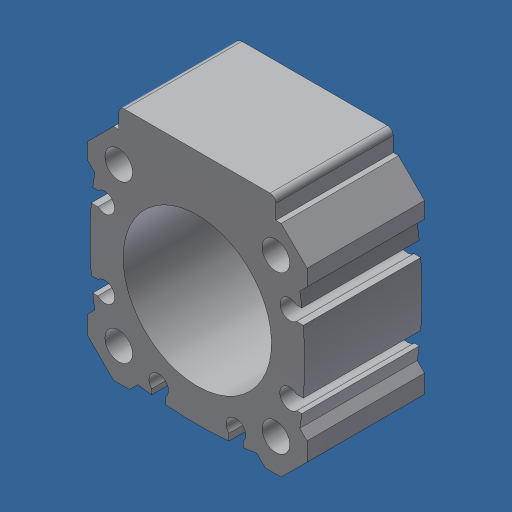
# Autodesk Inventor part: EXTRUSION, CYLINDER, ALUMINIUM, PHD, 32MM
Saved by Autodesk Inventor 2024.3 (Build 283343000, 343)
## iProperties
Manager: _
Category: _
Shininess: 64.0
Angle Display Precision: 2
Document Length Units: 11269
Document Angle Units: 11279
Document Time Units: 11290
Document Mass Units: 11286
Document Length Units Precision: 3
Document Angle Units Precision: 2
Part Number: EXTRUSION, CYLINDER, ALUMINIUM, PHD, 32MM
Material: Extrusion, Aluminum, PHD, 32MM
Document SubType Name: Modeling
Created: 2023-11-08
Designer: -
Manufacturer: Standard
Standards Organization: Custom
Checked By: 00
Engr Approved By: _
User Status: Work In Process
Description: EXTRUSION, CYLINDER, ALUMINIUM, PHD, 32MM
Density: 2.71 g/cm^3
Mass: 85.3878 g
Surface Area: 132.066 cm^2
Volume: 31.5084 cm^3
Mfg Approved By: Stephen.Oerton
Appearance: Aluminum - Flat
ILogicPurgeVersion: 2.2.20.20
OnSaveVersion: 2.2.20.20
Density: 0.0
Volumn: 0.0
Area: 0.0
PropertySet Name: Model Information
Control State: 0
Master: False
Checked Out: False
CN_MASS: 0.09
CN_SERVICEABLE: _
CL_runCount: 0
FIRST_DESCRIPTION: _
SECOND_DESCRIPTION: _
THIRD_DESCRIPTION: _
ModelCat: Uncategorized
Revision Number: A
Subject: _
Author: -
Keywords: -
Autodesk Inventor part; units mm, degrees
ref_plane "YZ Plane" through (0, 0, 0) normal (1, 0, 0) x (0, 1, 0)
ref_plane "XZ Plane" through (0, 0, 0) normal (0, 1, 0) x (-1, 0, 0)
ref_plane "XY Plane" through (0, 0, 0) normal (0, 0, 1) x (1, 0, 0)
sketch "Sketch1" plane through (0, 0, 0) normal (0, 0, 1) x (1, 0, 0)
  arc A0 (0, 16.053) -> (0, -16.053) centre (0, 0) ccw
  arc A1 (-15.7355, 27.991) -> (-17.0055, 26.721) centre (-15.7355, 26.721) ccw
  line L0 (-17.0055, 26.721) -> (-17.0055, 23.52)
  line L1 (-17.0055, 23.52) -> (-18.1469, 23.52)
  line L2 (0, 78.3044) -> (0, -31.8793) projected
  line L3 (-15.7355, 27.991) -> (0, 27.991)
  line L4 (-18.1469, 23.52) -> (-23.75, 17.9169)
  line L5 (-23.75, 17.9169) -> (-23.75, 14.428)
  line L6 (-23.75, 14.428) -> (-22.174, 12.852)
  line L7 (-22.6105, 9.8935) -> (-21.4771, 9.8935)
  arc A2 (-21.4771, 6.8205) -> (-21.4771, 9.8935) centre (-20.015, 8.357) ccw
  line L8 (-22.942, 6.8205) -> (-21.4771, 6.8205)
  arc A3 (-22.174, 12.852) -> (-22.6105, 9.8935) centre (54.6936, 0) ccw
  arc A4 (-21.544, -9.8935) -> (-21.544, -6.8205) centre (-20.015, -8.357) ccw
  line L9 (-22.942, -6.8205) -> (-21.544, -6.8205)
  line L10 (-22.6105, -9.8935) -> (-21.544, -9.8935)
  arc A5 (-22.942, 6.8205) -> (-22.942, -6.8205) centre (54.6936, 0) ccw
  arc A6 (-22.6105, -9.8935) -> (-22.174, -12.852) centre (54.6936, 0) ccw
  line L11 (-22.174, -12.852) -> (-23.75, -14.428)
  line L12 (-23.75, -14.428) -> (-23.75, -18.4059)
  line L13 (-23.75, -18.4059) -> (-18.1469, -24.009)
  line L14 (-18.1469, -24.009) -> (-14.687, -24.009)
  line L15 (-14.687, -24.009) -> (-12.852, -22.174)
  arc A7 (-6.8205, -21.4771) -> (-9.8935, -21.4771) centre (-8.357, -20.015) ccw
  line L16 (-9.8935, -21.4771) -> (-9.8935, -22.6105)
  line L17 (-6.8205, -21.4771) -> (-6.8205, -22.942)
  arc A8 (-12.852, -22.174) -> (-9.8935, -22.6105) centre (0, 54.6936) ccw
  arc A9 (-6.8205, -22.942) -> (0, -23.241) centre (0, 54.6936) ccw
  circle A10 centre (-17, -17) radius 3
  circle A11 centre (-17, 17) radius 3
  arc A12 (0, -16.053) -> (0, 16.053) centre (0, 0) ccw
  arc A13 (17.0055, 26.721) -> (15.7355, 27.991) centre (15.7355, 26.721) ccw
  line L18 (17.0055, 26.721) -> (17.0055, 23.52)
  line L19 (17.0055, 23.52) -> (18.1469, 23.52)
  line L20 (15.7355, 27.991) -> (0, 27.991)
  line L21 (18.1469, 23.52) -> (23.75, 17.9169)
  line L22 (23.75, 17.9169) -> (23.75, 14.428)
  line L23 (23.75, 14.428) -> (22.174, 12.852)
  line L24 (22.6105, 9.8935) -> (21.4771, 9.8935)
  arc A14 (21.4771, 9.8935) -> (21.4771, 6.8205) centre (20.015, 8.357) ccw
  line L25 (22.942, 6.8205) -> (21.4771, 6.8205)
  arc A15 (22.6105, 9.8935) -> (22.174, 12.852) centre (-54.6936, 0) ccw
  arc A16 (21.544, -6.8205) -> (21.544, -9.8935) centre (20.015, -8.357) ccw
  line L26 (22.942, -6.8205) -> (21.544, -6.8205)
  line L27 (22.6105, -9.8935) -> (21.544, -9.8935)
  arc A17 (22.942, -6.8205) -> (22.942, 6.8205) centre (-54.6936, 0) ccw
  arc A18 (22.174, -12.852) -> (22.6105, -9.8935) centre (-54.6936, 0) ccw
  line L28 (22.174, -12.852) -> (23.75, -14.428)
  line L29 (23.75, -14.428) -> (23.75, -18.4059)
  line L30 (23.75, -18.4059) -> (18.1469, -24.009)
  line L31 (18.1469, -24.009) -> (14.687, -24.009)
  line L32 (14.687, -24.009) -> (12.852, -22.174)
  arc A19 (9.8935, -21.4771) -> (6.8205, -21.4771) centre (8.357, -20.015) ccw
  line L33 (9.8935, -21.4771) -> (9.8935, -22.6105)
  line L34 (6.8205, -21.4771) -> (6.8205, -22.942)
  arc A20 (9.8935, -22.6105) -> (12.852, -22.174) centre (0, 54.6936) ccw
  arc A21 (0, -23.241) -> (6.8205, -22.942) centre (0, 54.6936) ccw
  circle A22 centre (17, -17) radius 3
  circle A23 centre (17, 17) radius 3
  arc A24 (22.174, -12.852) -> (22.6105, -9.8935) centre (-54.6936, 0) ccw
  arc A25 (22.942, -6.8205) -> (22.942, 6.8205) centre (-54.6936, 0) ccw
  dimension "d0" = 54.6936
  dimension "d2" = 54.6936
  dimension "d6" = 32.106
  dimension "d8" = 2.54
  dimension "d10" = 15.7355
  dimension "d11" = 26.721
  dimension "d12" = 18.1469
  dimension "d13" = 23.52
  dimension "d14" = 135
  dimension "d15" = 17.9169
  dimension "d16" = 3.4889
  dimension "d17" = 135
  dimension "d18" = 22.174
  dimension "d19" = 9.8935
  dimension "d22" = 22.6105
  dimension "d23" = 20.015
  dimension "d24" = 8.357
  dimension "d25" = 4.242
  dimension "d26" = 6.8205
  dimension "d27" = 8.357
  dimension "d28" = 4.3354
  dimension "d29" = 6.8205
  dimension "d30" = 9.8935
  dimension "d31" = 77.9346
  dimension "d32" = 22.174
  dimension "d33" = 12.852
  dimension "d34" = 45
  dimension "d35" = 14.428
  dimension "d37" = 18.4059
  dimension "d38" = 135
  dimension "d39" = 24.009
  dimension "d41" = 135
  dimension "d42" = 14.687
  dimension "d43" = 20.015
  dimension "d44" = 8.357
  dimension "d45" = 4.242
  dimension "d46" = 9.8935
  dimension "d47" = 6.8205
  dimension "d48" = 77.9346
  dimension "d49" = 77.9346
  dimension "d50" = 17
  dimension "d51" = 17
  dimension "d52" = 6
  dimension "d53" = 17
  dimension "d54" = 6
  constraints: 68 end point, 42 point on circle, 33 symmetric about line, 26 centre point, 6 perpendicular, 5 parallel, 4 point on line, 3 vertical alignment, 2 horizontal alignment, 2 tangent, 1 coincident, 1 horizontal, 29 other
  measures "d0" distance of A3.centre point (0, 0)
  measures "d2" distance of A8.centre point (0, 0)
  measures "d6" diameter of A0
  measures "d8" diameter of A1
  measures "d10" horizontal distance of point (0, 0) A1.centre
  measures "d11" vertical distance of point (0, 0) A1.centre
  measures "d12" distance from line of L1.end L2
  measures "d13" distance from line of point (0, 0) L1
  measures "d14" angle of L4 L1
  measures "d15" vertical distance of point (0, 0) L4.end
  measures "d16" distance of L4.end L5.end
  measures "d17" angle of L6 L5
  measures "d18" distance from line of L6.end L2
  measures "d19" distance from line of L7 point (0, 0)
  measures "d22" distance from line of L2 L7.start
  measures "d23" distance from line of L2 A2.centre
  measures "d24" vertical distance of A0.centre A2.centre
  measures "d25" diameter of A2
  measures "d26" distance from line of A0.centre L8
  measures "d27" vertical distance of point (0, 0) A4.centre
  measures "d28" diameter of A4
  measures "d29" distance from line of A0.centre L9
  measures "d30" distance from line of L10 point (0, 0)
  measures "d31" radius of A5
  measures "d32" distance from line of L2 L11.start
  measures "d33" vertical distance of L11.start A0.centre
  measures "d34" angle of L2 L11
  measures "d35" vertical distance of point (0, 0) L11.end
  measures "d37" vertical distance of point (0, 0) L12.end
  measures "d38" angle of L13 L12
  measures "d39" distance from line of point (0, 0) L14
  measures "d41" angle of L15 L14
  measures "d42" distance from line of L2 L14.end
  measures "d43" vertical distance of point (0, 0) A7.centre
  measures "d44" distance from line of L2 A7.centre
  measures "d45" diameter of A7
  measures "d46" distance between parallel lines of L2 L16
  measures "d47" distance between parallel lines of L2 L17
  measures "d48" radius of A9
  measures "d49" radius of A8
  measures "d50" distance from line of L2 A10.centre
  measures "d51" horizontal distance of A10.centre point (0, 0)
  measures "d52" diameter of A10
  measures "d53" horizontal distance of point (0, 0) A11.centre
  measures "d54" diameter of A11
extrude "PHD, 32MM" add sketch "Sketch1" against normal blind 25.4 contours A0 L2 A9 L17 A7 L16 A8 L15 L14 L13 L12 L11 A6 L10 A4 L9 A5 L8 A2 L7 A3 L6 L5 L4 L1 L0 A1 L3 | L2 L20 A13 L18 L19 L21 L22 L23 A15 L24 A14 L25 A17 L26 A16 L27 A18 L28 L29 L30 L31 L32 A20 L33 A19 L34 A21 A12
equation "\"d27\" = d24"
equation "\"d29\" = d26"
equation "\"d30\" = d19"
equation "\"d53\" = d51"
equation "\"d54\" = d52"
